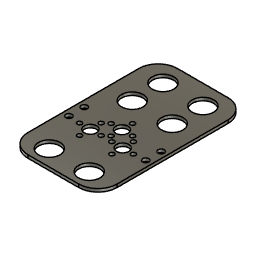
Robot assembly (Autodesk Fusion 360 archive; units mm, degrees)
design "base plate" references "Servo Bracket - U Shaped"
Autodesk Fusion 360 part; units mm, degrees
sketch "Sketch2" plane through (-1, 0, 0) normal (-1, 0, 0) x (0, -1, 0)
  line L0 (-8.755, -21) -> (-8.755, -25)
  circle A0 centre (-6.755, -25) radius 2
  line L1 (-8.755, -25) -> (-8.755, -29)
  line L2 (-8.755, -29) -> (7.245, -29)
  arc A1 (7.245, -29) -> (10.245, -26) centre (7.245, -26) ccw
  line L3 (10.245, -26) -> (10.245, -19.2)
  arc A2 (10.445, -19) -> (10.245, -19.2) centre (10.445, -19.2) ccw
  line L4 (10.445, -19) -> (15.745, -19)
  line L5 (15.745, -19) -> (15.745, 19)
  line L6 (15.745, 19) -> (10.445, 19)
  arc A3 (10.245, 19.2) -> (10.445, 19) centre (10.445, 19.2) ccw
  line L7 (10.245, 19.2) -> (10.245, 26)
  arc A4 (10.245, 26) -> (7.245, 29) centre (7.245, 26) ccw
  line L8 (7.245, 29) -> (-8.755, 29)
  line L9 (-8.755, 29) -> (-8.755, 25)
  circle A5 centre (-6.755, 25) radius 2
  line L10 (-8.755, 25) -> (-8.755, 21)
  line L11 (-8.755, 21) -> (-5.955, 21)
  arc A6 (-5.755, 20.8) -> (-5.955, 21) centre (-5.955, 20.8) ccw
  line L12 (-5.755, 20.8) -> (-5.755, 19.2)
  arc A7 (-5.955, 19) -> (-5.755, 19.2) centre (-5.955, 19.2) ccw
  line L13 (-5.955, 19) -> (-14.745, 19)
  arc A8 (-14.745, 19) -> (-17.745, 16) centre (-14.745, 16) ccw
  line L14 (-17.745, 16) -> (-17.745, -16)
  arc A9 (-17.745, -16) -> (-14.745, -19) centre (-14.745, -16) ccw
  line L15 (-14.745, -19) -> (-5.955, -19)
  arc A10 (-5.755, -19.2) -> (-5.955, -19) centre (-5.955, -19.2) ccw
  line L16 (-5.755, -19.2) -> (-5.755, -20.8)
  arc A11 (-5.955, -21) -> (-5.755, -20.8) centre (-5.955, -20.8) ccw
  line L17 (-5.955, -21) -> (-8.755, -21)
  circle A12 centre (-3.255, 10.5) radius 1.5
  circle A13 centre (10.745, 10.5) radius 1.5
  circle A14 centre (3.745, 3.5) radius 1.5
  circle A15 centre (3.745, 17.5) radius 1.5
  circle A16 centre (-13.255, 0) radius 1.5
  circle A17 centre (0.745, 0) radius 1.5
  circle A18 centre (-6.255, -7) radius 1.5
  circle A19 centre (-6.255, 7) radius 1.5
  circle A20 centre (-3.255, -10.5) radius 1.5
  circle A21 centre (10.745, -10.5) radius 1.5
  circle A22 centre (3.745, -17.5) radius 1.5
  circle A23 centre (3.745, -3.5) radius 1.5
  circle A24 centre (3.245, -25) radius 2
  circle A25 centre (3.245, 25) radius 2
  circle A26 centre (3.745, 10.5) radius 4
  circle A27 centre (-6.255, 0) radius 4
  circle A28 centre (3.745, -10.5) radius 4
  line L18 (-46.3299, -29) -> (25.8846, -29)
  line L19 (25.8846, 29) -> (-46.3299, 29)
  line L20 (-58.8299, 16.5) -> (-58.8299, -16.5)
  circle A29 centre (-6.755, -25) radius 2
  circle A30 centre (-13.255, 0) radius 1.5
  circle A31 centre (-6.255, 0) radius 4
  circle A32 centre (-6.255, -7) radius 1.5
  circle A33 centre (-3.255, -10.5) radius 1.5
  line L21 (-25, 0) -> (27.58, 0)
  circle A34 centre (-6.755, 25) radius 2
  circle A35 centre (-3.255, 10.5) radius 1.5
  circle A36 centre (-6.255, 7) radius 1.5
  circle A37 centre (3.245, -25) radius 2
  circle A38 centre (3.745, -17.5) radius 1.5
  circle A39 centre (3.745, -10.5) radius 4
  circle A40 centre (10.745, -10.5) radius 1.5
  circle A41 centre (3.745, -3.5) radius 1.5
  circle A42 centre (0.745, 0) radius 1.5
  circle A43 centre (3.245, 25) radius 2
  circle A44 centre (3.745, 17.5) radius 1.5
  circle A45 centre (3.745, 10.5) radius 4
  circle A46 centre (3.745, 3.5) radius 1.5
  circle A47 centre (-26, -13) radius 7
  circle A48 centre (-26, 13) radius 7
  circle A49 centre (28, -13) radius 7
  circle A50 centre (28, 13) radius 7
  line L22 (38.3846, -16.5) -> (38.3846, 16.5)
  arc A51 (-58.8299, -16.5) -> (-46.3299, -29) centre (-46.3299, -16.5) ccw
  arc A52 (-46.3299, 29) -> (-58.8299, 16.5) centre (-46.3299, 16.5) ccw
  arc A53 (25.8846, -29) -> (38.3846, -16.5) centre (25.8846, -16.5) ccw
  arc A54 (38.3846, 16.5) -> (25.8846, 29) centre (25.8846, 16.5) ccw
  circle A55 centre (-46, -13) radius 7
  circle A56 centre (-46, 13) radius 7
  point P0 (-58.8299, -29)
  point P1 (-58.8299, 29)
  point P2 (10.745, 10.5)
  dimension "d2" = 58
  dimension "d4" = 14
  dimension "d5" = 14
  dimension "d11" = 12.5
  dimension "d12" = 12.5
  dimension "d13" = 12.5
  dimension "d16" = -20
  dimension "d17" = 0
  constraint horizontal L18
  constraint horizontal L19
  constraint vertical L20
  constraint collinear L2 L18
  constraint concentric A0 A29
  constraint concentric A16 A30
  constraint concentric A27 A31
  constraint concentric A18 A32
  constraint concentric A20 A33
  constraint perpendicular L14 L21
  constraint symmetric A29 L21 A34
  constraint symmetric A32 L21 A36
  constraint symmetric A33 L21 A35
  constraint concentric A24 A37
  constraint concentric A22 A38
  constraint concentric A28 A39
  constraint concentric A21 A40
  constraint concentric A23 A41
  constraint concentric A17 A42
  constraint symmetric L21 A37 A43
  constraint symmetric L21 A38 A44
  constraint symmetric L21 A39 A45
  constraint symmetric L21 A21.centre P2
  constraint symmetric L21 A41 A46
  constraint symmetric L21 A47 A48
  constraint symmetric L21 A49 A50
  constraint perpendicular L19 L22
  constraint coincident P0 L18
  constraint coincident P0 L20
  constraint tangent L18 A51
  constraint tangent L20 A51
  constraint coincident P1 L20
  constraint coincident P1 L19
  constraint tangent L20 A52
  constraint tangent L19 A52
  constraint tangent L18 A53
  constraint tangent L22 A53
  constraint tangent L22 A54
  constraint tangent L19 A54
  constraint equal A53 A54
  measures "d2" distance of P0 P1
  measures "d4" diameter of A47
  measures "d5" diameter of A49
  measures "d11" radius of A51
  measures "d12" radius of A52
  measures "d13" radius of A53
extrude "Extrude1" add sketch "Sketch2" along normal blind 2 contours L0 L1 L2 A1 L3 A2 L4 L5 L14 A9 L15 A10 L16 A11 L17 A16 A17 A27 L18 A30 A31 L21 A42 | L0 L1 L9 L10 L11 A6 L12 A7 L13 A8 L14 A9 L15 A10 L16 A11 L17 L18 L19 L20 A51 A52 | A1 L3 A2 L4 L5 L6 A3 L7 A4 L18 L19 L22 A53 A54 | L5 L6 A3 L7 A4 L8 L9 L10 L11 A6 L12 A7 L13 A8 L14 A16 A17 A27 L19 A30 A31 L21 A42
move_body "Move1" bodies 1 to x (0, 0, 1) y (0, 1, 0) z (-1, 0, 0) at (-0.4047, 0, 3.1428)
